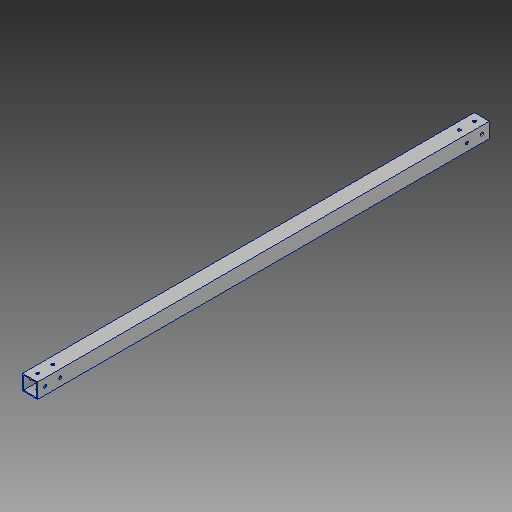
# Autodesk Inventor part: 1x1
Saved by Autodesk Inventor 2018 (Build 220112000, 112)
## iProperties
Created: 2018-06-29
Part Number: 1x1
Material: Aluminum 6061
Document SubType Name: Modeling
Designer: s-2512711
Density: 2.7 g/cm^3
Appearance: Aluminum - Flat
Author: s-2512711
Autodesk Inventor part; units mm, degrees
ref_plane "YZ Plane" through (0, 0, 0) normal (1, 0, 0) x (0, 1, 0)
ref_plane "XZ Plane" through (0, 0, 0) normal (0, 1, 0) x (-1, 0, 0)
ref_plane "XY Plane" through (0, 0, 0) normal (0, 0, 1) x (1, 0, 0)
sketch "Sketch1" plane through (0, 0, 0) normal (0, 0, 1) x (1, 0, 0)
  line L0 (0, 0) -> (25.4, 0)
  line L1 (25.4, 0) -> (25.4, 25.4)
  line L2 (25.4, 25.4) -> (0, 25.4)
  line L3 (0, 25.4) -> (0, 0)
  line L4 (1.5875, 23.8125) -> (23.8125, 23.8125)
  line L5 (23.8125, 23.8125) -> (23.8125, 1.5875)
  line L6 (23.8125, 1.5875) -> (1.5875, 1.5875)
  line L7 (1.5875, 1.5875) -> (1.5875, 23.8125)
  dimension "d0" = 25.4
  dimension "d1" = 25.4
  dimension "d2" = 1.5875
  dimension "d3" = 1.5875
  dimension "d4" = 1.5875
  dimension "d5" = 1.5875
  constraints: 16 end point, 4 parallel, 2 horizontal, 2 perpendicular
  measures "d0" distance of L2.end L1.end
  measures "d1" distance of L1.end L0.end
  measures "d2" distance between parallel lines of L2 L4
  measures "d3" distance between parallel lines of L1 L5
  measures "d4" distance between parallel lines of L3 L7
  measures "d5" distance between parallel lines of L0 L6
extrude "Extrusion1" add sketch "Sketch1" along normal blind 762
sketch "Sketch2" plane through (25.4, 0, 0) normal (1, 0, 0) x (0, 0, -1)
  line L0 (0, 1.5875) -> (0, 23.8125) projected
  line L1 (0, 12.7) -> (-762, 12.7)
  line L2 (-762, 23.8125) -> (-762, 1.5875) projected
  line L3 (-762, 12.7) -> (-749.3, 12.7)
  line L4 (-749.3, 12.7) -> (-723.9, 12.7)
  line L5 (0, 12.7) -> (-12.7, 12.7)
  line L6 (-12.7, 12.7) -> (-38.1, 12.7)
  circle A0 centre (-12.7, 12.7) radius 2.54
  circle A1 centre (-38.1, 12.7) radius 2.54
  circle A2 centre (-723.9, 12.7) radius 2.54
  circle A3 centre (-749.3, 12.7) radius 2.54
  point P0 (0, 0)
  dimension "d8" = 12.7
  dimension "d9" = 25.4
  dimension "d10" = 12.7
  dimension "d11" = 25.4
  dimension "d12" = 5.08
  constraints: 10 end point, 4 centre point, 4 coincident, 4 point on line, 2 midpoint
  measures "d8" distance of L1.end L3.end
  measures "d9" distance of L3.end L4.end
  measures "d10" distance of L1.start L5.end
  measures "d11" distance of L5.end L6.end
  measures "d12" diameter of A0
extrude "Extrusion2" cut sketch "Sketch2" against normal blind 25.4
sketch "Sketch3" plane through (0, 25.4, 0) normal (0, 1, 0) x (1, 0, 0)
  line L0 (23.8125, 0) -> (1.5875, 0) projected
  line L1 (12.7, 0) -> (12.7, -762)
  line L2 (25.4, -762) -> (0, -762) projected
  line L3 (12.7, -762) -> (12.7, -749.3)
  line L4 (12.7, -749.3) -> (12.7, -723.9)
  line L5 (12.7, 0) -> (12.7, -12.7)
  line L6 (12.7, -12.7) -> (12.7, -38.1)
  circle A0 centre (12.7, -12.7) radius 2.54
  circle A1 centre (12.7, -38.1) radius 2.54
  circle A2 centre (12.7, -723.9) radius 2.54
  circle A3 centre (12.7, -749.3) radius 2.54
  point P0 (0, 0)
  dimension "d15" = 12.7
  dimension "d16" = 25.4
  dimension "d17" = 12.7
  dimension "d18" = 25.4
  dimension "d19" = 5.08
  constraints: 10 end point, 4 centre point, 4 coincident, 4 point on line, 2 midpoint
  measures "d15" distance of L1.end L3.end
  measures "d16" distance of L3.end L4.end
  measures "d17" distance of L1.start L5.end
  measures "d18" distance of L5.end L6.end
  measures "d19" diameter of A0
extrude "Extrusion3" cut sketch "Sketch3" against normal blind 25.4
body "Solid1"
